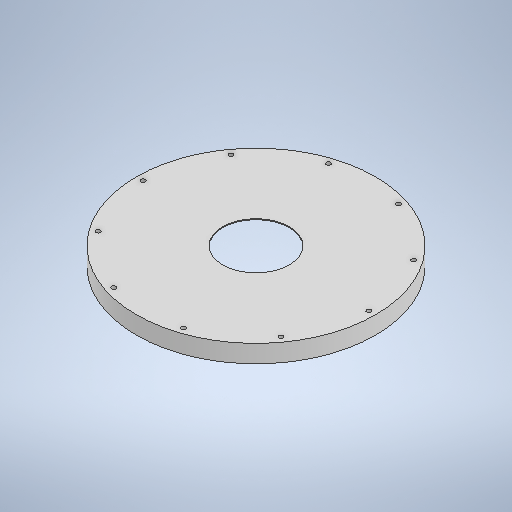
# Autodesk Inventor part: Cylinder Spacer (x3)
Saved by Autodesk Inventor 2025 (Build 290162000, 162)
## iProperties
Created: 2024-04-28
Part Number: Cylinder Spacer (x3)
Material: Generic
Document SubType Name: Modeling
Designer: Thienan Hoang
Density: 1 g/cm^3
Appearance: Default
Author: Thienan Hoang
Autodesk Inventor part; units mm, degrees
ref_plane "YZ Plane" through (0, 0, 0) normal (1, 0, 0) x (0, 1, 0)
ref_plane "XZ Plane" through (0, 0, 0) normal (0, 1, 0) x (-1, 0, 0)
ref_plane "XY Plane" through (0, 0, 0) normal (0, 0, 1) x (1, 0, 0)
sketch "Sketch1" plane through (0, 0, 0) normal (0, 1, 0) x (-1, 0, 0)
  circle A0 centre (0, 0) radius 135
  circle A1 centre (0, 0) radius 110
  dimension "d0" = 270
  dimension "d1" = 220
  constraints: 2 centre point, 2 coincident
  measures "d0" diameter of A0
  measures "d1" diameter of A1
extrude "Extrusion1" add sketch "Sketch1" along normal mid plane 20
sketch "Sketch2" plane through (0, 10, 0) normal (0, 1, 0) x (1, 0, 0)
  circle A0 centre (0, 0) radius 37.5
  circle A1 centre (0, 0) radius 135
  dimension "d4" = 75
  dimension "d20" = 270
  constraints: 2 centre point, 2 coincident
  measures "d4" diameter of A0
  measures "d20" diameter of A1
extrude "Extrusion2" add sketch "Sketch2" against normal blind 1
sketch "Sketch3" plane through (0, 10, 0) normal (0, 1, 0) x (1, 0, 0)
  circle A0 centre (0, 0) radius 127.5
  circle A1 centre (127.5, 0) radius 2.5
  circle A2 centre (103.1497, 74.9426) radius 2.5
  circle A3 centre (39.3997, 121.2597) radius 2.5
  circle A4 centre (-39.3997, 121.2597) radius 2.5
  circle A5 centre (-103.1497, 74.9426) radius 2.5
  circle A6 centre (-127.5, 0) radius 2.5
  circle A7 centre (-103.1497, -74.9426) radius 2.5
  circle A8 centre (-39.3997, -121.2597) radius 2.5
  circle A9 centre (39.3997, -121.2597) radius 2.5
  circle A10 centre (103.1497, -74.9426) radius 2.5
  dimension "d7" = 255
  dimension "d8" = 5
  dimension "d11" = 360
  constraints: 10 centre point, 1 coincident, 1 horizontal alignment, 23 other
  measures "d8" diameter of A1
hole "Hole1" at (127.5, 10, 0) at (103.1497, 10, 74.9426) at (39.3997, 10, 121.2597) at (-39.3997, 10, 121.2597) at (-103.1497, 10, 74.9426) at (-127.5, 10, 0) at (-103.1497, 10, -74.9426) at (-39.3997, 10, -121.2597) at (39.3997, 10, -121.2597) at (103.1497, 10, -74.9426) direction (0, -1, 0) diameter 5 end through all
body "Solid1"
